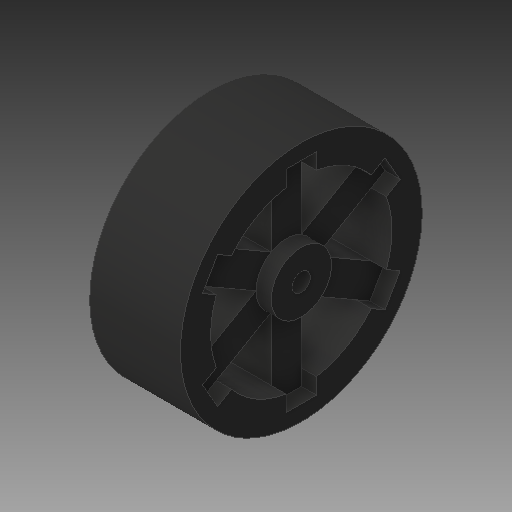
# Autodesk Inventor part: Part3
Saved by Autodesk Inventor 2019 (Build 230136000, 136)
## iProperties
Created: 2019-08-08
Part Number: Part3
Material: Rubber
Document SubType Name: Modeling
Designer: daozhou.cen
Density: 0.93 g/cm^3
Appearance: Rubber - Black
Author: daozhou.cen
Autodesk Inventor part; units mm, degrees
ref_plane "YZ Plane" through (0, 0, 0) normal (1, 0, 0) x (0, 1, 0)
ref_plane "XZ Plane" through (0, 0, 0) normal (0, 1, 0) x (-1, 0, 0)
ref_plane "XY Plane" through (0, 0, 0) normal (0, 0, 1) x (1, 0, 0)
sketch "Sketch1" plane through (0, 0, 0) normal (1, 0, 0) x (0, 1, 0)
  circle A0 centre (0, 0) radius 20
  circle A1 centre (0, 0) radius 15
  circle A2 centre (0, 0) radius 5
  line L0 (20, 0) -> (9.9317, 0) construction
  line L1 (9.9317, 0) -> (0, 0) construction
  line L2 (17.4317, -2.5) -> (2.4317, -2.5)
  line L3 (2.4317, -2.5) -> (2.4317, 2.5)
  line L4 (2.4317, 2.5) -> (17.4317, 2.5)
  line L5 (17.4317, 2.5) -> (17.4317, -2.5)
  line L6 (17.4317, -2.5) -> (2.4317, 2.5) construction
  line L7 (2.4317, -2.5) -> (17.4317, 2.5) construction
  line L8 (-0.9492, 3.3559) -> (6.5508, 16.3463)
  line L9 (10.8809, 13.8463) -> (3.3809, 0.8559)
  line L10 (6.5508, 16.3463) -> (10.8809, 13.8463)
  line L11 (3.3809, 0.8559) -> (-0.9492, 3.3559)
  line L12 (-3.3809, 0.8559) -> (-10.8809, 13.8463)
  line L13 (-6.5508, 16.3463) -> (0.9492, 3.3559)
  line L14 (-10.8809, 13.8463) -> (-6.5508, 16.3463)
  line L15 (0.9492, 3.3559) -> (-3.3809, 0.8559)
  line L16 (-2.4317, -2.5) -> (-17.4317, -2.5)
  line L17 (-17.4317, 2.5) -> (-2.4317, 2.5)
  line L18 (-17.4317, -2.5) -> (-17.4317, 2.5)
  line L19 (-2.4317, 2.5) -> (-2.4317, -2.5)
  line L20 (0.9492, -3.3559) -> (-6.5508, -16.3463)
  line L21 (-10.8809, -13.8463) -> (-3.3809, -0.8559)
  line L22 (-6.5508, -16.3463) -> (-10.8809, -13.8463)
  line L23 (-3.3809, -0.8559) -> (0.9492, -3.3559)
  line L24 (3.3809, -0.8559) -> (10.8809, -13.8463)
  line L25 (6.5508, -16.3463) -> (-0.9492, -3.3559)
  line L26 (10.8809, -13.8463) -> (6.5508, -16.3463)
  line L27 (-0.9492, -3.3559) -> (3.3809, -0.8559)
  dimension "d0" = 40
  dimension "d1" = 30
  dimension "d2" = 10
  dimension "d4" = 15
  dimension "d5" = 5
  dimension "d8" = 360
  constraints: 56 end point, 3 coincident, 3 horizontal, 2 centre point, 2 midpoint, 2 parallel, 1 horizontal alignment, 1 perpendicular, 51 other
  measures "d1" diameter of A1
  measures "d2" diameter of A2
  measures "d4" distance of L3.end L4.end
  measures "d5" distance of L2.end L3.end
extrude "Extrusion1" add sketch "Sketch1" along normal mid plane 15 contours A0 | L4 L3 L11 L15 L13 A2 | L9 L11 L3 L4 | A2 L24 L27 L3 L11 L9 | A2 L20 L23 L27 L3 L2 | L2 L3 L27 L24 | L8 L11 L15 L19 L17 A2 | L13 L15 L11 L8 | L25 L27 L23 L20 | A2 L16 L19 L23 L27 L25 | L12 L15 L19 L23 L21 A2 | L17 L19 L15 L12 | L3 L27 L23 L19 L15 L11 | L21 L23 L19 L16
extrude "Extrusion2" add sketch "Sketch1" along normal mid plane 10 contours A1 L2 A2 L4 | A1 L4 L5 L2 | L9 A2 L8 A1 | A1 L8 L10 L9 | L4 L3 L11 L15 L13 A2 | L9 L11 L3 L4 | A2 L24 L27 L3 L11 L9 | L24 L26 L25 A1 | A1 L25 A2 L24 | A2 L20 L23 L27 L3 L2 | L2 L3 L27 L24 | L8 L11 L15 L19 L17 A2 | L13 L15 L11 L8 | A2 L12 A1 L13 | L20 A1 L21 A2 | L25 L27 L23 L20 | A2 L16 L19 L23 L27 L25 | A1 L12 L14 L13 | L12 L15 L19 L23 L21 A2 | L17 L19 L15 L12 | A2 L16 A1 L17 | L20 L22 L21 A1 | L21 L23 L19 L16 | A1 L16 L18 L17
sketch "Sketch2" plane through (-7.5, 0, 0) normal (-1, 0, 0) x (0, 0, 1)
  circle A0 centre (0, 0) radius 1.5
  dimension "d14" = 3
  constraints: 1 centre point, 1 coincident
  measures "d14" diameter of A0
extrude "Extrusion3" cut sketch "Sketch2" against normal up to next
body "Solid1"
